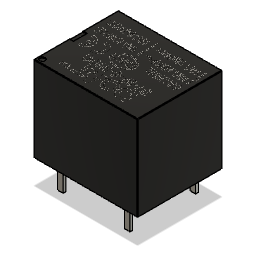
Doat-5volt Relay v1 (Autodesk Fusion 360 design; units mm, degrees)
Autodesk Fusion 360 part; units mm, degrees
sketch "Sketch1" plane through (0, 0, 0) normal (0, 1, 0) x (1, 0, 0)
  line L0 (9.5, -7.75) -> (-9.5, -7.75)
  line L1 (-9.5, -7.75) -> (-9.5, 7.75)
  line L2 (-9.5, 7.75) -> (9.5, 7.75)
  line L3 (9.5, 7.75) -> (9.5, -7.75)
  line L4 (9.5, -7.75) -> (-9.5, 7.75) construction
  line L5 (-9.5, -7.75) -> (9.5, 7.75) construction
  dimension "d1" = 19
  dimension "d2" = 15.5
  constraint horizontal L0
  constraint perpendicular L0 L1
  constraint parallel L0 L2
  constraint parallel L1 L3
  constraint coincident L4 origin
  constraint coincident L5 origin
  measures "d1" distance of L1.end L2.end
  measures "d2" distance of L0.end L1.end
extrude "Extrude1" add sketch "Sketch1" along normal blind 15.5
fillet "Fillet1" radius 0.1 4 edges at (-9.5, 7.75, -7.75) (9.5, 7.75, -7.75) (9.5, 7.75, 7.75) (-9.5, 7.75, 7.75) 1 faces at (3.1667, 15.5, 2.5833)
sketch "Sketch2" plane through (0, 0, 0) normal (0, -1, 0) x (1, 0, 0)
  arc A0 (9.5, 7.65) -> (9.4, 7.75) centre (9.4, 7.65) ccw
  line L0 (9.4, 7.75) -> (-9.4, 7.75)
  arc A1 (-9.4, 7.75) -> (-9.5, 7.65) centre (-9.4, 7.65) ccw
  line L1 (-9.5, 7.65) -> (-9.5, -7.65)
  arc A2 (-9.5, -7.65) -> (-9.4, -7.75) centre (-9.4, -7.65) ccw
  line L2 (-9.4, -7.75) -> (9.4, -7.75)
  arc A3 (9.4, -7.75) -> (9.5, -7.65) centre (9.4, -7.65) ccw
  line L3 (9.5, -7.65) -> (9.5, 7.65)
  line L4 (6.1, 6) -> (-6.1, 6) construction
  line L5 (-6.1, 6) -> (-6.1, -6) construction
  line L6 (-6.1, -6) -> (6.1, -6) construction
  line L7 (6.1, -6) -> (6.1, 6) construction
  line L8 (6.1, 6) -> (-6.1, -6) construction
  line L9 (-6.1, 6) -> (6.1, -6) construction
  line L10 (-6.1, 0) -> (-8.1, 0) construction
  line L11 (-5.6, 5.75) -> (-6.6, 5.75)
  line L12 (-6.6, 5.75) -> (-6.6, 6.25)
  line L13 (-6.6, 6.25) -> (-5.6, 6.25)
  line L14 (-5.6, 6.25) -> (-5.6, 5.75)
  line L15 (-5.6, 5.75) -> (-6.6, 6.25) construction
  line L16 (-6.6, 5.75) -> (-5.6, 6.25) construction
  line L17 (-5.6, -5.75) -> (-6.6, -5.75)
  line L18 (-6.6, -5.75) -> (-6.6, -6.25)
  line L19 (-6.6, -6.25) -> (-5.6, -6.25)
  line L20 (-5.6, -6.25) -> (-5.6, -5.75)
  line L21 (-5.6, -5.75) -> (-6.6, -6.25) construction
  line L22 (-6.6, -5.75) -> (-5.6, -6.25) construction
  line L23 (6.6, 6.25) -> (5.6, 6.25)
  line L24 (5.6, 6.25) -> (5.6, 5.75)
  line L25 (5.6, 5.75) -> (6.6, 5.75)
  line L26 (6.6, 5.75) -> (6.6, 6.25)
  line L27 (6.6, 6.25) -> (5.6, 5.75) construction
  line L28 (5.6, 6.25) -> (6.6, 5.75) construction
  line L29 (6.6, -5.75) -> (5.6, -5.75)
  line L30 (5.6, -5.75) -> (5.6, -6.25)
  line L31 (5.6, -6.25) -> (6.6, -6.25)
  line L32 (6.6, -6.25) -> (6.6, -5.75)
  line L33 (6.6, -5.75) -> (5.6, -6.25) construction
  line L34 (5.6, -5.75) -> (6.6, -6.25) construction
  line L35 (-7.85, -0.5) -> (-8.35, -0.5)
  line L36 (-8.35, -0.5) -> (-8.35, 0.5)
  line L37 (-8.35, 0.5) -> (-7.85, 0.5)
  line L38 (-7.85, 0.5) -> (-7.85, -0.5)
  line L39 (-7.85, -0.5) -> (-8.35, 0.5) construction
  line L40 (-8.35, -0.5) -> (-7.85, 0.5) construction
  point P0 (-6.1, 6)
  point P1 (-6.1, -6)
  point P2 (6.1, 6)
  point P3 (6.1, -6)
  point P4 (-8.1, 0)
  dimension "d7" = 12.2
  dimension "d8" = 12
  dimension "d9" = 2
  dimension "d10" = 1
  dimension "d11" = 0.5
  dimension "d12" = 1
  dimension "d13" = 0.5
  dimension "d14" = 1
  dimension "d15" = 0.5
  dimension "d16" = 1
  dimension "d17" = 0.5
  dimension "d18" = 0.5
  dimension "d19" = 1
  constraint horizontal L4
  constraint perpendicular L4 L5
  constraint parallel L4 L6
  constraint parallel L5 L7
  constraint coincident L8 origin
  constraint coincident L9 origin
  constraint midpoint L5 L10.start
  constraint perpendicular L5 L10
  constraint horizontal L11
  constraint perpendicular L11 L12
  constraint parallel L11 L13
  constraint parallel L12 L14
  constraint coincident L15 P0
  constraint coincident L16 P0
  constraint coincident P0 L4.end
  constraint horizontal L17
  constraint perpendicular L17 L18
  constraint parallel L17 L19
  constraint parallel L18 L20
  constraint coincident L21 P1
  constraint coincident L22 P1
  constraint coincident P1 L5.end
  constraint horizontal L23
  constraint perpendicular L23 L24
  constraint parallel L23 L25
  constraint parallel L24 L26
  constraint coincident L27 P2
  constraint coincident L28 P2
  constraint coincident P2 L4.start
  constraint horizontal L29
  constraint perpendicular L29 L30
  constraint parallel L29 L31
  constraint parallel L30 L32
  constraint coincident L33 P3
  constraint coincident L34 P3
  constraint coincident P3 L6.end
  constraint horizontal L35
  constraint perpendicular L35 L36
  constraint parallel L35 L37
  constraint parallel L36 L38
  constraint coincident L39 P4
  constraint coincident L40 P4
  constraint coincident P4 L10.end
  measures "d7" distance of P1 P3
  measures "d8" distance of P0 P1
  measures "d9" distance of L10.start P4
  measures "d10" distance of L12.end L13.end
  measures "d11" distance of L11.end L12.end
  measures "d12" distance of L18.end L19.end
  measures "d13" distance of L17.end L18.end
  measures "d14" distance of L24.end L25.end
  measures "d15" distance of L23.end L24.end
  measures "d16" distance of L30.end L31.end
  measures "d17" distance of L29.end L30.end
  measures "d18" distance of L36.end L37.end
  measures "d19" distance of L35.end L36.end
extrude "Extrude2" add sketch "Sketch2" along normal blind 4.5 contours L11 L12 L13 L14 | L17 L18 L19 L20 | L23 L24 L25 L26 | L29 L30 L31 L32 | L35 L36 L37 L38
sketch "Sketch3" plane through (0, 0, 0) normal (0, -1, 0) x (1, 0, 0)
  line L0 (6.6, -6.25) -> (5.6, -6.25)
  line L1 (5.6, -6.25) -> (5.6, -5.75)
  line L2 (5.6, -5.75) -> (6.6, -5.75)
  line L3 (6.6, -5.75) -> (6.6, -6.25)
  line L4 (-5.6, -6.25) -> (-6.6, -6.25)
  line L5 (-6.6, -6.25) -> (-6.6, -5.75)
  line L6 (-6.6, -5.75) -> (-5.6, -5.75)
  line L7 (-5.6, -5.75) -> (-5.6, -6.25)
  line L8 (6.6, 5.75) -> (5.6, 5.75)
  line L9 (5.6, 5.75) -> (5.6, 6.25)
  line L10 (5.6, 6.25) -> (6.6, 6.25)
  line L11 (6.6, 6.25) -> (6.6, 5.75)
  line L12 (-7.85, 0.5) -> (-7.85, -0.5)
  line L13 (-7.85, -0.5) -> (-8.35, -0.5)
  line L14 (-8.35, -0.5) -> (-8.35, 0.5)
  line L15 (-8.35, 0.5) -> (-7.85, 0.5)
  line L16 (-5.6, 6.25) -> (-5.6, 5.75)
  line L17 (-5.6, 5.75) -> (-6.6, 5.75)
  line L18 (-6.6, 5.75) -> (-6.6, 6.25)
  line L19 (-6.6, 6.25) -> (-5.6, 6.25)
  arc A0 (9.5, 7.65) -> (9.4, 7.75) centre (9.4, 7.65) ccw
  line L20 (9.4, 7.75) -> (-9.4, 7.75)
  arc A1 (-9.4, 7.75) -> (-9.5, 7.65) centre (-9.4, 7.65) ccw
  line L21 (-9.5, 7.65) -> (-9.5, -7.65)
  arc A2 (-9.5, -7.65) -> (-9.4, -7.75) centre (-9.4, -7.65) ccw
  line L22 (-9.4, -7.75) -> (9.4, -7.75)
  arc A3 (9.4, -7.75) -> (9.5, -7.65) centre (9.4, -7.65) ccw
  line L23 (9.5, -7.65) -> (9.5, 7.65)
  circle A4 centre (-6.5, 0) radius 0.65
  dimension "d22" = 1.3
  measures "d22" diameter of A4
extrude "Extrude3" cut sketch "Sketch3" against normal blind 0.1 contours A4
sketch "Sketch4" plane through (0, 0.1, 0) normal (0, -1, 0) x (1, 0, 0)
  circle A0 centre (-6.5, 0) radius 0.65
  circle A1 centre (-6.5, 0) radius 0.15
  dimension "d25" = 0.3
  constraint concentric A0 A1
  measures "d25" diameter of A1
extrude "Extrude4" add sketch "Sketch4" along normal blind 0.1 contours A1
sketch "Sketch5" plane through (0, 15.5, 0) normal (0, 1, 0) x (-1, 0, 0)
  line L0 (9.4, 7.65) -> (-9.4, 7.65)
  line L1 (-9.4, 7.65) -> (-9.4, -7.65)
  line L2 (-9.4, -7.65) -> (9.4, -7.65)
  line L3 (9.4, -7.65) -> (9.4, 7.65)
  line L4 (10.1, 1.25) -> (8.7, 1.25)
  line L5 (8.7, 1.25) -> (8.7, -1.25)
  line L6 (8.7, -1.25) -> (10.1, -1.25)
  line L7 (10.1, -1.25) -> (10.1, 1.25)
  line L8 (10.1, 1.25) -> (8.7, -1.25) construction
  line L9 (8.7, 1.25) -> (10.1, -1.25) construction
  point P0 (9.4, 0)
  dimension "d28" = 1.4
  dimension "d29" = 2.5
  constraint horizontal L4
  constraint perpendicular L4 L5
  constraint parallel L4 L6
  constraint parallel L5 L7
  constraint coincident L8 P0
  constraint coincident L9 P0
  constraint midpoint L3 P0
  measures "d28" distance of L5.end L6.end
  measures "d29" distance of L4.end L5.end
extrude "Extrude5" cut sketch "Sketch5" against normal blind 0.2 contours L3 L4 L6 L7 | L3 L4 L5 L6
sketch "Sketch6" plane through (0, 15.5, 0) normal (0, 1, 0) x (-1, 0, 0)
  line L0 (8.7, 1.25) -> (9.4, 1.25)
  line L1 (9.4, 1.25) -> (9.4, 7.65)
  line L2 (9.4, 7.65) -> (-9.4, 7.65)
  line L3 (-9.4, 7.65) -> (-9.4, -7.65)
  line L4 (-9.4, -7.65) -> (9.4, -7.65)
  line L5 (9.4, -7.65) -> (9.4, -1.25)
  line L6 (9.4, -1.25) -> (8.7, -1.25)
  line L7 (8.7, -1.25) -> (8.7, 1.25)
  circle A0 centre (8.725, 6.9131) radius 0.5
  dimension "d32" = 1
  measures "d32" diameter of A0
extrude "Extrude6" cut sketch "Sketch6" against normal blind 0.2 contours A0
